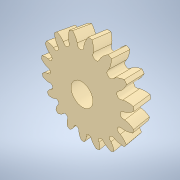
# Autodesk Inventor part: Промежуточная шестерня (малая)
Saved by Autodesk Inventor 2021.1 (Build 251245010, 245A)
## iProperties
Created: 2026-04-13
Part Number: Промежуточная шестерня (малая)
Material: Generic
Document SubType Name: Modeling
Designer: Андрей Тарасов
Density: 1 g/cm^3
Appearance: Default
Author: Андрей Тарасов
Autodesk Inventor part; units mm, degrees
ref_plane "YZ Plane" through (0, 0, 0) normal (1, 0, 0) x (0, 1, 0)
ref_plane "XZ Plane" through (0, 0, 0) normal (0, 1, 0) x (-1, 0, 0)
ref_plane "XY Plane" through (0, 0, 0) normal (0, 0, 1) x (1, 0, 0)
sketch "Sketch1" plane through (0, 0, 0) normal (0, 0, 1) x (1, 0, 0)
  spline S0 degree 3 poles (-2.4677, 16.4029) (-2.3891, 16.3117) (-2.2319, 16.1291) (-2.0115, 15.8426) (-1.8036, 15.5469) (-1.6113, 15.2408) (-1.4365, 14.9243) (-1.3084, 14.6515) (-1.219, 14.4277) (-1.1604, 14.2569) (-1.1092, 14.0833) (-1.0894, 13.9644) (-1.0796, 13.905) knots 0 0 0 0 0.036134 0.072267 0.1084 0.144533 0.180664 0.216793 0.23486 0.252926 0.270991 0.289046 0.289046 0.289046 0.289046
  spline S1 degree 3 poles (-1.0796, 13.905) (-1.0738, 13.8258) (-1.0651, 13.707) (-1.0412, 13.55) (-1.0167, 13.4334) (-0.9834, 13.319) (-0.9444, 13.2063) (-0.8925, 13.099) (-0.8339, 12.9952) (-0.7615, 12.9003) (-0.6769, 12.8161) (-0.5801, 12.7461) (-0.473, 12.6931) (-0.3574, 12.6608) (-0.1982, 12.6537) (0, 12.6626) (0.1982, 12.6537) (0.3574, 12.6608) (0.473, 12.6931) (0.5801, 12.7461) (0.6769, 12.8161) (0.7615, 12.9003) (0.8339, 12.9952) (0.8925, 13.099) (0.9444, 13.2063) (0.9834, 13.319) (1.0167, 13.4334) (1.0412, 13.55) (1.0651, 13.707) (1.0738, 13.8258) (1.0796, 13.905) knots 0 0 0 0 0.023807 0.035713 0.047621 0.059527 0.071434 0.083337 0.095237 0.107137 0.119035 0.130931 0.142823 0.154717 0.166615 0.19043 0.214245 0.226143 0.238037 0.249929 0.261825 0.273723 0.285623 0.297523 0.309426 0.321333 0.333239 0.345147 0.357054 0.38086 0.38086 0.38086 0.38086
  spline S2 degree 3 poles (1.0796, 13.905) (1.0894, 13.9644) (1.1092, 14.0833) (1.1604, 14.2569) (1.219, 14.4277) (1.3084, 14.6515) (1.4365, 14.9243) (1.6113, 15.2408) (1.8036, 15.5469) (2.0115, 15.8426) (2.2319, 16.1291) (2.3891, 16.3117) (2.4677, 16.4029) knots 0 0 0 0 0.018055 0.03612 0.054187 0.072254 0.108383 0.144514 0.180646 0.216779 0.252913 0.289046 0.289046 0.289046 0.289046
  circle A0 centre (0, 0) radius 12.659 construction
  circle A1 centre (0, 0) radius 13.946 construction
  circle A2 centre (0, 0) radius 14.841 construction
  circle A3 centre (0, 0) radius 16.5875
  spline S3 degree 3 poles (-6.0297, 12.5761) (-5.9957, 12.5043) (-5.9447, 12.3967) (-5.8658, 12.2589) (-5.8008, 12.159) (-5.7284, 12.0644) (-5.6513, 11.9734) (-5.5642, 11.8921) (-5.472, 11.8164) (-5.3702, 11.7541) (-5.2609, 11.7061) (-5.1453, 11.6758) (-5.0263, 11.6651) (-4.9069, 11.6767) (-4.7559, 11.7276) (-4.5743, 11.8075) (-4.3862, 11.8708) (-4.2403, 11.9349) (-4.1443, 12.0068) (-4.0635, 12.0949) (-3.9985, 12.1951) (-3.9501, 12.3043) (-3.9168, 12.4189) (-3.8996, 12.5369) (-3.89, 12.6557) (-3.8944, 12.7749) (-3.9046, 12.8935) (-3.9239, 13.0112) (-3.9584, 13.1662) (-3.9932, 13.2801) (-4.0164, 13.356) knots 0 0 0 0 0.023807 0.035713 0.047621 0.059527 0.071434 0.083337 0.095237 0.107137 0.119035 0.130931 0.142823 0.154717 0.166615 0.19043 0.214245 0.226143 0.238037 0.249929 0.261825 0.273723 0.285623 0.297523 0.309426 0.321333 0.333239 0.345147 0.357054 0.38086 0.38086 0.38086 0.38086
  spline S4 degree 3 poles (-4.0164, 13.356) (-4.0287, 13.415) (-4.0532, 13.533) (-4.0682, 13.7133) (-4.0752, 13.8938) (-4.0727, 14.1348) (-4.0517, 14.4354) (-4.0031, 14.7937) (-3.9343, 15.1486) (-3.8474, 15.4994) (-3.7453, 15.8462) (-3.6647, 16.0732) (-3.6243, 16.1867) knots 0 0 0 0 0.018055 0.03612 0.054187 0.072254 0.108383 0.144514 0.180646 0.216779 0.252913 0.289046 0.289046 0.289046 0.289046
  spline S5 degree 3 poles (-8.2265, 14.4038) (-8.1202, 14.3471) (-7.9077, 14.2337) (-7.5986, 14.0461) (-7.298, 13.8455) (-7.0081, 13.6295) (-6.7308, 13.3975) (-6.5128, 13.1895) (-6.3486, 13.0131) (-6.2322, 12.875) (-6.1218, 12.7316) (-6.0604, 12.6279) (-6.0297, 12.5761) knots 0 0 0 0 0.036134 0.072267 0.1084 0.144533 0.180664 0.216793 0.23486 0.252926 0.270991 0.289046 0.289046 0.289046 0.289046
  spline S6 degree 3 poles (-10.1655, 9.5486) (-10.1079, 9.494) (-10.0215, 9.4121) (-9.8981, 9.3121) (-9.8014, 9.2424) (-9.6997, 9.1804) (-9.595, 9.1233) (-9.4844, 9.079) (-9.3711, 9.0418) (-9.2536, 9.0204) (-9.1344, 9.0151) (-9.0156, 9.0287) (-8.9008, 9.0617) (-8.7936, 9.1156) (-8.6712, 9.2176) (-8.5307, 9.3578) (-8.3782, 9.4847) (-8.2654, 9.5972) (-8.2018, 9.699) (-8.1583, 9.8102) (-8.1339, 9.9272) (-8.1281, 10.0465) (-8.1385, 10.1654) (-8.1652, 10.2816) (-8.1991, 10.3959) (-8.2462, 10.5054) (-8.2986, 10.6124) (-8.3591, 10.7151) (-8.4473, 10.8472) (-8.5209, 10.9408) (-8.5699, 11.0032) knots 0 0 0 0 0.023807 0.035713 0.047621 0.059527 0.071434 0.083337 0.095237 0.107137 0.119035 0.130931 0.142823 0.154717 0.166615 0.19043 0.214245 0.226143 0.238037 0.249929 0.261825 0.273723 0.285623 0.297523 0.309426 0.321333 0.333239 0.345147 0.357054 0.38086 0.38086 0.38086 0.38086
  spline S7 degree 3 poles (-8.5699, 11.0032) (-8.6027, 11.0538) (-8.6682, 11.1549) (-8.7473, 11.3177) (-8.819, 11.4835) (-8.9037, 11.7091) (-8.9928, 11.997) (-9.0769, 12.3486) (-9.141, 12.7044) (-9.1866, 13.0629) (-9.2167, 13.4232) (-9.2235, 13.664) (-9.2269, 13.7844) knots 0 0 0 0 0.018055 0.03612 0.054187 0.072254 0.108383 0.144514 0.180646 0.216779 0.252913 0.289046 0.289046 0.289046 0.289046
  spline S8 degree 3 poles (-12.8743, 10.4594) (-12.7547, 10.4449) (-12.5155, 10.4159) (-12.1596, 10.3527) (-11.8067, 10.2742) (-11.4584, 10.1775) (-11.116, 10.0614) (-10.8376, 9.9461) (-10.6208, 9.841) (-10.4623, 9.7542) (-10.3076, 9.6604) (-10.2129, 9.5859) (-10.1655, 9.5486) knots 0 0 0 0 0.036134 0.072267 0.1084 0.144533 0.180664 0.216793 0.23486 0.252926 0.270991 0.289046 0.289046 0.289046 0.289046
  spline S9 degree 3 poles (-12.9285, 5.2316) (-12.855, 5.2015) (-12.7448, 5.1563) (-12.5936, 5.1077) (-12.4783, 5.0776) (-12.361, 5.0565) (-12.2428, 5.0411) (-12.1236, 5.0398) (-12.0046, 5.046) (-11.8873, 5.0685) (-11.7742, 5.1066) (-11.6684, 5.1622) (-11.5732, 5.2344) (-11.4928, 5.3234) (-11.4155, 5.4628) (-11.3351, 5.6442) (-11.2387, 5.8177) (-11.1741, 5.9633) (-11.1516, 6.0812) (-11.1513, 6.2007) (-11.1707, 6.3186) (-11.2085, 6.4318) (-11.2611, 6.539) (-11.3279, 6.6377) (-11.4009, 6.732) (-11.4844, 6.8171) (-11.5719, 6.8979) (-11.6654, 6.9718) (-11.7953, 7.0632) (-11.8977, 7.1239) (-11.9661, 7.1644) knots 0 0 0 0 0.023807 0.035713 0.047621 0.059527 0.071434 0.083337 0.095237 0.107137 0.119035 0.130931 0.142823 0.154717 0.166615 0.19043 0.214245 0.226143 0.238037 0.249929 0.261825 0.273723 0.285623 0.297523 0.309426 0.321333 0.333239 0.345147 0.357054 0.38086 0.38086 0.38086 0.38086
  spline S10 degree 3 poles (-11.9661, 7.1644) (-12.0148, 7.1997) (-12.1125, 7.2704) (-12.245, 7.3935) (-12.3718, 7.5222) (-12.5323, 7.702) (-12.7194, 7.9383) (-12.9247, 8.2358) (-13.113, 8.5444) (-13.2851, 8.8622) (-13.4433, 9.1873) (-13.5367, 9.4094) (-13.5833, 9.5204) knots 0 0 0 0 0.018055 0.03612 0.054187 0.072254 0.108383 0.144514 0.180646 0.216779 0.252913 0.289046 0.289046 0.289046 0.289046
  spline S11 degree 3 poles (-15.7833, 5.1024) (-15.6665, 5.1321) (-15.433, 5.1914) (-15.0783, 5.2611) (-14.7209, 5.3153) (-14.3612, 5.351) (-14, 5.3664) (-13.6987, 5.3595) (-13.4585, 5.3398) (-13.2794, 5.3161) (-13.1013, 5.2846) (-12.986, 5.2493) (-12.9285, 5.2316) knots 0 0 0 0 0.036134 0.072267 0.1084 0.144533 0.180664 0.216793 0.23486 0.252926 0.270991 0.289046 0.289046 0.289046 0.289046
  spline S12 degree 3 poles (-13.9453, 0.208) (-13.8659, 0.2065) (-13.7468, 0.2042) (-13.5883, 0.2134) (-13.4699, 0.2271) (-13.353, 0.2497) (-13.2371, 0.2781) (-13.1255, 0.3199) (-13.0167, 0.3687) (-12.9156, 0.4321) (-12.8238, 0.5085) (-12.7452, 0.5985) (-12.6826, 0.7002) (-12.6397, 0.8123) (-12.618, 0.9701) (-12.6086, 1.1684) (-12.5814, 1.3649) (-12.5738, 1.5241) (-12.5953, 1.6421) (-12.6382, 1.7536) (-12.6989, 1.8566) (-12.775, 1.9485) (-12.8628, 2.0294) (-12.9608, 2.0974) (-13.0629, 2.1589) (-13.1715, 2.2081) (-13.2823, 2.2519) (-13.3961, 2.287) (-13.5503, 2.3253) (-13.6678, 2.3449) (-13.7461, 2.3579) knots 0 0 0 0 0.023807 0.035713 0.047621 0.059527 0.071434 0.083337 0.095237 0.107137 0.119035 0.130931 0.142823 0.154717 0.166615 0.19043 0.214245 0.226143 0.238037 0.249929 0.261825 0.273723 0.285623 0.297523 0.309426 0.321333 0.333239 0.345147 0.357054 0.38086 0.38086 0.38086 0.38086
  spline S13 degree 3 poles (-13.7461, 2.3579) (-13.8043, 2.3733) (-13.9209, 2.4039) (-14.089, 2.4709) (-14.2537, 2.5451) (-14.4683, 2.6547) (-14.7281, 2.8074) (-15.0271, 3.0107) (-15.3141, 3.2304) (-15.5894, 3.4646) (-15.8544, 3.7106) (-16.0216, 3.884) (-16.1053, 3.9707) knots 0 0 0 0 0.018055 0.03612 0.054187 0.072254 0.108383 0.144514 0.180646 0.216779 0.252913 0.289046 0.289046 0.289046 0.289046
  spline S14 degree 3 poles (-16.5607, -0.9437) (-16.4625, -0.8739) (-16.2662, -0.7342) (-15.9606, -0.5411) (-15.647, -0.3614) (-15.3244, -0.1982) (-14.9932, -0.0534) (-14.7097, 0.049) (-14.4787, 0.1174) (-14.3031, 0.16) (-14.1256, 0.195) (-14.0054, 0.2037) (-13.9453, 0.208) knots 0 0 0 0 0.036134 0.072267 0.1084 0.144533 0.180664 0.216793 0.23486 0.252926 0.270991 0.289046 0.289046 0.289046 0.289046
  spline S15 degree 3 poles (-13.0788, -4.8436) (-13.0042, -4.8164) (-12.8923, -4.7755) (-12.7478, -4.7096) (-12.6423, -4.6541) (-12.5415, -4.5908) (-12.4437, -4.5225) (-12.3547, -4.4432) (-12.2709, -4.3584) (-12.1995, -4.2628) (-12.1416, -4.1584) (-12.1008, -4.046) (-12.0791, -3.9285) (-12.0796, -3.8086) (-12.1164, -3.6535) (-12.1792, -3.4653) (-12.2249, -3.2722) (-12.2753, -3.121) (-12.338, -3.0187) (-12.4182, -2.9302) (-12.5121, -2.8562) (-12.6163, -2.7979) (-12.7274, -2.7542) (-12.8432, -2.7262) (-12.9607, -2.7057) (-13.0797, -2.6991) (-13.1988, -2.6983) (-13.3177, -2.7066) (-13.4753, -2.7267) (-13.5919, -2.7508) (-13.6696, -2.7669) knots 0 0 0 0 0.023807 0.035713 0.047621 0.059527 0.071434 0.083337 0.095237 0.107137 0.119035 0.130931 0.142823 0.154717 0.166615 0.19043 0.214245 0.226143 0.238037 0.249929 0.261825 0.273723 0.285623 0.297523 0.309426 0.321333 0.333239 0.345147 0.357054 0.38086 0.38086 0.38086 0.38086
  spline S16 degree 3 poles (-13.6696, -2.7669) (-13.7295, -2.7737) (-13.8492, -2.7872) (-14.0302, -2.7855) (-14.2106, -2.7758) (-14.4503, -2.7511) (-14.7477, -2.7025) (-15.0999, -2.621) (-15.447, -2.5198) (-15.7883, -2.4009) (-16.1242, -2.2672) (-16.3428, -2.166) (-16.4521, -2.1153) knots 0 0 0 0 0.018055 0.03612 0.054187 0.072254 0.108383 0.144514 0.180646 0.216779 0.252913 0.289046 0.289046 0.289046 0.289046
  spline S17 degree 3 poles (-15.1014, -6.8624) (-15.0352, -6.7618) (-14.9026, -6.5606) (-14.6873, -6.2702) (-14.4598, -5.9894) (-14.218, -5.7206) (-13.9614, -5.4659) (-13.7341, -5.2681) (-13.5434, -5.1208) (-13.3951, -5.0176) (-13.2421, -4.9209) (-13.1332, -4.8694) (-13.0788, -4.8436) knots 0 0 0 0 0.036134 0.072267 0.1084 0.144533 0.180664 0.216793 0.23486 0.252926 0.270991 0.289046 0.289046 0.289046 0.289046
  spline S18 degree 3 poles (-10.4459, -9.2411) (-10.3862, -9.1888) (-10.2966, -9.1103) (-10.1857, -8.9966) (-10.1074, -8.9068) (-10.0362, -8.8113) (-9.9697, -8.7123) (-9.9154, -8.6062) (-9.8679, -8.4969) (-9.8358, -8.3819) (-9.8195, -8.2636) (-9.822, -8.1441) (-9.8443, -8.0267) (-9.8881, -7.915) (-9.9784, -7.7837) (-10.105, -7.6309) (-10.2173, -7.4673) (-10.3189, -7.3446) (-10.4144, -7.2719) (-10.5211, -7.2183) (-10.6354, -7.1832) (-10.7536, -7.1665) (-10.873, -7.1659) (-10.9911, -7.1817) (-11.108, -7.2049) (-11.2214, -7.2418) (-11.3328, -7.2841) (-11.4406, -7.3348) (-11.5803, -7.4104) (-11.6803, -7.475) (-11.747, -7.5181) knots 0 0 0 0 0.023807 0.035713 0.047621 0.059527 0.071434 0.083337 0.095237 0.107137 0.119035 0.130931 0.142823 0.154717 0.166615 0.19043 0.214245 0.226143 0.238037 0.249929 0.261825 0.273723 0.285623 0.297523 0.309426 0.321333 0.333239 0.345147 0.357054 0.38086 0.38086 0.38086 0.38086
  spline S19 degree 3 poles (-11.747, -7.5181) (-11.8004, -7.5461) (-11.9072, -7.6019) (-12.0765, -7.6657) (-12.2482, -7.7218) (-12.4807, -7.7854) (-12.7755, -7.8475) (-13.1334, -7.8988) (-13.4936, -7.9298) (-13.8548, -7.9421) (-14.2163, -7.9388) (-14.4567, -7.9234) (-14.577, -7.9157) knots 0 0 0 0 0.018055 0.03612 0.054187 0.072254 0.108383 0.144514 0.180646 0.216779 0.252913 0.289046 0.289046 0.289046 0.289046
  spline S20 degree 3 poles (-11.6027, -11.8543) (-11.5772, -11.7365) (-11.5263, -11.501) (-11.4305, -11.1525) (-11.3197, -10.8084) (-11.1914, -10.4705) (-11.0441, -10.1403) (-10.9036, -9.8737) (-10.7789, -9.6675) (-10.6779, -9.5177) (-10.5703, -9.3722) (-10.4873, -9.2848) (-10.4459, -9.2411) knots 0 0 0 0 0.036134 0.072267 0.1084 0.144533 0.180664 0.216793 0.23486 0.252926 0.270991 0.289046 0.289046 0.289046 0.289046
  spline S21 degree 3 poles (-6.4022, -12.3906) (-6.3654, -12.3202) (-6.3103, -12.2147) (-6.2479, -12.0686) (-6.2073, -11.9565) (-6.1755, -11.8418) (-6.1493, -11.7254) (-6.1369, -11.6069) (-6.1321, -11.4878) (-6.1437, -11.3689) (-6.1712, -11.2528) (-6.2168, -11.1423) (-6.28, -11.0409) (-6.3611, -10.9526) (-6.4928, -10.8627) (-6.666, -10.7659) (-6.8298, -10.654) (-6.9689, -10.5762) (-7.0842, -10.5429) (-7.2031, -10.5316) (-7.3223, -10.5401) (-7.4386, -10.5672) (-7.5501, -10.6098) (-7.6546, -10.6672) (-7.7552, -10.7311) (-7.8477, -10.8064) (-7.9362, -10.8861) (-8.0184, -10.9723) (-8.1214, -11.0933) (-8.1913, -11.1897) (-8.2379, -11.254) knots 0 0 0 0 0.023807 0.035713 0.047621 0.059527 0.071434 0.083337 0.095237 0.107137 0.119035 0.130931 0.142823 0.154717 0.166615 0.19043 0.214245 0.226143 0.238037 0.249929 0.261825 0.273723 0.285623 0.297523 0.309426 0.321333 0.333239 0.345147 0.357054 0.38086 0.38086 0.38086 0.38086
  spline S22 degree 3 poles (-8.2379, -11.254) (-8.2776, -11.2993) (-8.357, -11.39) (-8.4918, -11.5106) (-8.6317, -11.625) (-8.8255, -11.7682) (-9.078, -11.9326) (-9.3932, -12.1097) (-9.7178, -12.2687) (-10.0502, -12.4107) (-10.3885, -12.5383) (-10.6183, -12.6107) (-10.7331, -12.647) knots 0 0 0 0 0.018055 0.03612 0.054187 0.072254 0.108383 0.144514 0.180646 0.216779 0.252913 0.289046 0.289046 0.289046 0.289046
  spline S23 degree 3 poles (-6.5369, -15.2451) (-6.5557, -15.1262) (-6.5933, -14.8882) (-6.6299, -14.5285) (-6.6509, -14.1677) (-6.6533, -13.8062) (-6.6353, -13.4451) (-6.6006, -13.1458) (-6.5588, -12.9084) (-6.5187, -12.7323) (-6.4709, -12.5578) (-6.4251, -12.4463) (-6.4022, -12.3906) knots 0 0 0 0 0.036134 0.072267 0.1084 0.144533 0.180664 0.216793 0.23486 0.252926 0.270991 0.289046 0.289046 0.289046 0.289046
  spline S24 degree 3 poles (-1.4939, -13.8666) (-1.485, -13.7877) (-1.4717, -13.6694) (-1.4663, -13.5106) (-1.469, -13.3915) (-1.4807, -13.2729) (-1.4983, -13.155) (-1.5296, -13.04) (-1.5681, -12.9272) (-1.6219, -12.8206) (-1.6895, -12.7222) (-1.7719, -12.6356) (-1.8675, -12.5639) (-1.9751, -12.5109) (-2.1302, -12.4747) (-2.3267, -12.447) (-2.52, -12.4018) (-2.6777, -12.3795) (-2.7973, -12.3901) (-2.9123, -12.4225) (-3.0203, -12.4735) (-3.1189, -12.5408) (-3.2076, -12.6207) (-3.2843, -12.712) (-3.355, -12.8079) (-3.414, -12.9116) (-3.4678, -13.0178) (-3.5133, -13.128) (-3.5656, -13.2779) (-3.596, -13.3931) (-3.6162, -13.4699) knots 0 0 0 0 0.023807 0.035713 0.047621 0.059527 0.071434 0.083337 0.095237 0.107137 0.119035 0.130931 0.142823 0.154717 0.166615 0.19043 0.214245 0.226143 0.238037 0.249929 0.261825 0.273723 0.285623 0.297523 0.309426 0.321333 0.333239 0.345147 0.357054 0.38086 0.38086 0.38086 0.38086
  spline S25 degree 3 poles (-3.6162, -13.4699) (-3.6368, -13.5265) (-3.6781, -13.6397) (-3.7603, -13.8009) (-3.8494, -13.9581) (-3.9784, -14.1616) (-4.1544, -14.4062) (-4.3843, -14.6852) (-4.6296, -14.9507) (-4.8883, -15.2032) (-5.1576, -15.4444) (-5.3457, -15.5949) (-5.4397, -15.6702) knots 0 0 0 0 0.018055 0.03612 0.054187 0.072254 0.108383 0.144514 0.180646 0.216779 0.252913 0.289046 0.289046 0.289046 0.289046
  spline S26 degree 3 poles (-0.5883, -16.5771) (-0.6488, -16.4729) (-0.7698, -16.2646) (-0.9339, -15.9424) (-1.0838, -15.6136) (-1.2166, -15.2773) (-1.3303, -14.9341) (-1.406, -14.6425) (-1.4528, -14.4061) (-1.4791, -14.2273) (-1.4975, -14.0473) (-1.4951, -13.9268) (-1.4939, -13.8666) knots 0 0 0 0 0.036134 0.072267 0.1084 0.144533 0.180664 0.216793 0.23486 0.252926 0.270991 0.289046 0.289046 0.289046 0.289046
  spline S27 degree 3 poles (3.6162, -13.4699) (3.596, -13.3931) (3.5656, -13.2779) (3.5133, -13.128) (3.4678, -13.0178) (3.414, -12.9116) (3.355, -12.8079) (3.2843, -12.712) (3.2076, -12.6207) (3.1189, -12.5408) (3.0203, -12.4735) (2.9123, -12.4225) (2.7973, -12.3901) (2.6777, -12.3795) (2.52, -12.4018) (2.3267, -12.447) (2.1302, -12.4747) (1.9751, -12.5109) (1.8675, -12.5639) (1.7719, -12.6356) (1.6895, -12.7222) (1.6219, -12.8206) (1.5681, -12.9272) (1.5296, -13.04) (1.4983, -13.155) (1.4807, -13.2729) (1.469, -13.3915) (1.4663, -13.5106) (1.4717, -13.6694) (1.485, -13.7877) (1.4939, -13.8666) knots 0 0 0 0 0.023807 0.035713 0.047621 0.059527 0.071434 0.083337 0.095237 0.107137 0.119035 0.130931 0.142823 0.154717 0.166615 0.19043 0.214245 0.226143 0.238037 0.249929 0.261825 0.273723 0.285623 0.297523 0.309426 0.321333 0.333239 0.345147 0.357054 0.38086 0.38086 0.38086 0.38086
  spline S28 degree 3 poles (1.4939, -13.8666) (1.4951, -13.9268) (1.4975, -14.0473) (1.4791, -14.2273) (1.4528, -14.4061) (1.406, -14.6425) (1.3303, -14.9341) (1.2166, -15.2773) (1.0838, -15.6136) (0.9339, -15.9424) (0.7698, -16.2646) (0.6488, -16.4729) (0.5883, -16.5771) knots 0 0 0 0 0.018055 0.03612 0.054187 0.072254 0.108383 0.144514 0.180646 0.216779 0.252913 0.289046 0.289046 0.289046 0.289046
  spline S29 degree 3 poles (5.4397, -15.6702) (5.3457, -15.5949) (5.1576, -15.4444) (4.8883, -15.2032) (4.6296, -14.9507) (4.3843, -14.6852) (4.1544, -14.4062) (3.9784, -14.1616) (3.8494, -13.9581) (3.7603, -13.8009) (3.6781, -13.6397) (3.6368, -13.5265) (3.6162, -13.4699) knots 0 0 0 0 0.036134 0.072267 0.1084 0.144533 0.180664 0.216793 0.23486 0.252926 0.270991 0.289046 0.289046 0.289046 0.289046
  spline S30 degree 3 poles (8.2379, -11.254) (8.1913, -11.1897) (8.1214, -11.0933) (8.0184, -10.9723) (7.9362, -10.8861) (7.8477, -10.8064) (7.7552, -10.7311) (7.6546, -10.6672) (7.5501, -10.6098) (7.4386, -10.5672) (7.3223, -10.5401) (7.2031, -10.5316) (7.0842, -10.5429) (6.9689, -10.5762) (6.8298, -10.654) (6.666, -10.7659) (6.4928, -10.8627) (6.3611, -10.9526) (6.28, -11.0409) (6.2168, -11.1423) (6.1712, -11.2528) (6.1437, -11.3689) (6.1321, -11.4878) (6.1369, -11.6069) (6.1493, -11.7254) (6.1755, -11.8418) (6.2073, -11.9565) (6.2479, -12.0686) (6.3103, -12.2147) (6.3654, -12.3202) (6.4022, -12.3906) knots 0 0 0 0 0.023807 0.035713 0.047621 0.059527 0.071434 0.083337 0.095237 0.107137 0.119035 0.130931 0.142823 0.154717 0.166615 0.19043 0.214245 0.226143 0.238037 0.249929 0.261825 0.273723 0.285623 0.297523 0.309426 0.321333 0.333239 0.345147 0.357054 0.38086 0.38086 0.38086 0.38086
  spline S31 degree 3 poles (6.4022, -12.3906) (6.4251, -12.4463) (6.4709, -12.5578) (6.5187, -12.7323) (6.5588, -12.9084) (6.6006, -13.1458) (6.6353, -13.4451) (6.6533, -13.8062) (6.6509, -14.1677) (6.6299, -14.5285) (6.5933, -14.8882) (6.5557, -15.1262) (6.5369, -15.2451) knots 0 0 0 0 0.018055 0.03612 0.054187 0.072254 0.108383 0.144514 0.180646 0.216779 0.252913 0.289046 0.289046 0.289046 0.289046
  spline S32 degree 3 poles (10.7331, -12.647) (10.6183, -12.6107) (10.3885, -12.5383) (10.0502, -12.4107) (9.7178, -12.2687) (9.3932, -12.1097) (9.078, -11.9326) (8.8255, -11.7682) (8.6317, -11.625) (8.4918, -11.5106) (8.357, -11.39) (8.2776, -11.2993) (8.2379, -11.254) knots 0 0 0 0 0.036134 0.072267 0.1084 0.144533 0.180664 0.216793 0.23486 0.252926 0.270991 0.289046 0.289046 0.289046 0.289046
  spline S33 degree 3 poles (11.747, -7.5181) (11.6803, -7.475) (11.5803, -7.4104) (11.4406, -7.3348) (11.3328, -7.2841) (11.2214, -7.2418) (11.108, -7.2049) (10.9911, -7.1817) (10.873, -7.1659) (10.7536, -7.1665) (10.6354, -7.1832) (10.5211, -7.2183) (10.4144, -7.2719) (10.3189, -7.3446) (10.2173, -7.4673) (10.105, -7.6309) (9.9784, -7.7837) (9.8881, -7.915) (9.8443, -8.0267) (9.822, -8.1441) (9.8195, -8.2636) (9.8358, -8.3819) (9.8679, -8.4969) (9.9154, -8.6062) (9.9697, -8.7123) (10.0362, -8.8113) (10.1074, -8.9068) (10.1857, -8.9966) (10.2966, -9.1103) (10.3862, -9.1888) (10.4459, -9.2411) knots 0 0 0 0 0.023807 0.035713 0.047621 0.059527 0.071434 0.083337 0.095237 0.107137 0.119035 0.130931 0.142823 0.154717 0.166615 0.19043 0.214245 0.226143 0.238037 0.249929 0.261825 0.273723 0.285623 0.297523 0.309426 0.321333 0.333239 0.345147 0.357054 0.38086 0.38086 0.38086 0.38086
  spline S34 degree 3 poles (10.4459, -9.2411) (10.4873, -9.2848) (10.5703, -9.3722) (10.6779, -9.5177) (10.7789, -9.6675) (10.9036, -9.8737) (11.0441, -10.1403) (11.1914, -10.4705) (11.3197, -10.8084) (11.4305, -11.1525) (11.5263, -11.501) (11.5772, -11.7365) (11.6027, -11.8543) knots 0 0 0 0 0.018055 0.03612 0.054187 0.072254 0.108383 0.144514 0.180646 0.216779 0.252913 0.289046 0.289046 0.289046 0.289046
  spline S35 degree 3 poles (14.577, -7.9157) (14.4567, -7.9234) (14.2163, -7.9388) (13.8548, -7.9421) (13.4936, -7.9298) (13.1334, -7.8988) (12.7755, -7.8475) (12.4807, -7.7854) (12.2482, -7.7218) (12.0765, -7.6657) (11.9072, -7.6019) (11.8004, -7.5461) (11.747, -7.5181) knots 0 0 0 0 0.036134 0.072267 0.1084 0.144533 0.180664 0.216793 0.23486 0.252926 0.270991 0.289046 0.289046 0.289046 0.289046
  spline S36 degree 3 poles (13.6696, -2.7669) (13.5919, -2.7508) (13.4753, -2.7267) (13.3177, -2.7066) (13.1988, -2.6983) (13.0797, -2.6991) (12.9607, -2.7057) (12.8432, -2.7262) (12.7274, -2.7542) (12.6163, -2.7979) (12.5121, -2.8562) (12.4182, -2.9302) (12.338, -3.0187) (12.2753, -3.121) (12.2249, -3.2722) (12.1792, -3.4653) (12.1164, -3.6535) (12.0796, -3.8086) (12.0791, -3.9285) (12.1008, -4.046) (12.1416, -4.1584) (12.1995, -4.2628) (12.2709, -4.3584) (12.3547, -4.4432) (12.4437, -4.5225) (12.5415, -4.5908) (12.6423, -4.6541) (12.7478, -4.7096) (12.8923, -4.7755) (13.0042, -4.8164) (13.0788, -4.8436) knots 0 0 0 0 0.023807 0.035713 0.047621 0.059527 0.071434 0.083337 0.095237 0.107137 0.119035 0.130931 0.142823 0.154717 0.166615 0.19043 0.214245 0.226143 0.238037 0.249929 0.261825 0.273723 0.285623 0.297523 0.309426 0.321333 0.333239 0.345147 0.357054 0.38086 0.38086 0.38086 0.38086
  spline S37 degree 3 poles (13.0788, -4.8436) (13.1332, -4.8694) (13.2421, -4.9209) (13.3951, -5.0176) (13.5434, -5.1208) (13.7341, -5.2681) (13.9614, -5.4659) (14.218, -5.7206) (14.4598, -5.9894) (14.6873, -6.2702) (14.9026, -6.5606) (15.0352, -6.7618) (15.1014, -6.8624) knots 0 0 0 0 0.018055 0.03612 0.054187 0.072254 0.108383 0.144514 0.180646 0.216779 0.252913 0.289046 0.289046 0.289046 0.289046
  spline S38 degree 3 poles (16.4521, -2.1153) (16.3428, -2.166) (16.1242, -2.2672) (15.7883, -2.4009) (15.447, -2.5198) (15.0999, -2.621) (14.7477, -2.7025) (14.4503, -2.7511) (14.2106, -2.7758) (14.0302, -2.7855) (13.8492, -2.7872) (13.7295, -2.7737) (13.6696, -2.7669) knots 0 0 0 0 0.036134 0.072267 0.1084 0.144533 0.180664 0.216793 0.23486 0.252926 0.270991 0.289046 0.289046 0.289046 0.289046
  spline S39 degree 3 poles (13.7461, 2.3579) (13.6678, 2.3449) (13.5503, 2.3253) (13.3961, 2.287) (13.2823, 2.2519) (13.1715, 2.2081) (13.0629, 2.1589) (12.9608, 2.0974) (12.8628, 2.0294) (12.775, 1.9485) (12.6989, 1.8566) (12.6382, 1.7536) (12.5953, 1.6421) (12.5738, 1.5241) (12.5814, 1.3649) (12.6086, 1.1684) (12.618, 0.9701) (12.6397, 0.8123) (12.6826, 0.7002) (12.7452, 0.5985) (12.8238, 0.5085) (12.9156, 0.4321) (13.0167, 0.3687) (13.1255, 0.3199) (13.2371, 0.2781) (13.353, 0.2497) (13.4699, 0.2271) (13.5883, 0.2134) (13.7468, 0.2042) (13.8659, 0.2065) (13.9453, 0.208) knots 0 0 0 0 0.023807 0.035713 0.047621 0.059527 0.071434 0.083337 0.095237 0.107137 0.119035 0.130931 0.142823 0.154717 0.166615 0.19043 0.214245 0.226143 0.238037 0.249929 0.261825 0.273723 0.285623 0.297523 0.309426 0.321333 0.333239 0.345147 0.357054 0.38086 0.38086 0.38086 0.38086
  spline S40 degree 3 poles (13.9453, 0.208) (14.0054, 0.2037) (14.1256, 0.195) (14.3031, 0.16) (14.4787, 0.1174) (14.7097, 0.049) (14.9932, -0.0534) (15.3244, -0.1982) (15.647, -0.3614) (15.9606, -0.5411) (16.2662, -0.7342) (16.4625, -0.8739) (16.5607, -0.9437) knots 0 0 0 0 0.018055 0.03612 0.054187 0.072254 0.108383 0.144514 0.180646 0.216779 0.252913 0.289046 0.289046 0.289046 0.289046
  spline S41 degree 3 poles (16.1053, 3.9707) (16.0216, 3.884) (15.8544, 3.7106) (15.5894, 3.4646) (15.3141, 3.2304) (15.0271, 3.0107) (14.7281, 2.8074) (14.4683, 2.6547) (14.2537, 2.5451) (14.089, 2.4709) (13.9209, 2.4039) (13.8043, 2.3733) (13.7461, 2.3579) knots 0 0 0 0 0.036134 0.072267 0.1084 0.144533 0.180664 0.216793 0.23486 0.252926 0.270991 0.289046 0.289046 0.289046 0.289046
  spline S42 degree 3 poles (11.9661, 7.1644) (11.8977, 7.1239) (11.7953, 7.0632) (11.6654, 6.9718) (11.5719, 6.8979) (11.4844, 6.8171) (11.4009, 6.732) (11.3279, 6.6377) (11.2611, 6.539) (11.2085, 6.4318) (11.1707, 6.3186) (11.1513, 6.2007) (11.1516, 6.0812) (11.1741, 5.9633) (11.2387, 5.8177) (11.3351, 5.6442) (11.4155, 5.4628) (11.4928, 5.3234) (11.5732, 5.2344) (11.6684, 5.1622) (11.7742, 5.1066) (11.8873, 5.0685) (12.0046, 5.046) (12.1236, 5.0398) (12.2428, 5.0411) (12.361, 5.0565) (12.4783, 5.0776) (12.5936, 5.1077) (12.7448, 5.1563) (12.855, 5.2015) (12.9285, 5.2316) knots 0 0 0 0 0.023807 0.035713 0.047621 0.059527 0.071434 0.083337 0.095237 0.107137 0.119035 0.130931 0.142823 0.154717 0.166615 0.19043 0.214245 0.226143 0.238037 0.249929 0.261825 0.273723 0.285623 0.297523 0.309426 0.321333 0.333239 0.345147 0.357054 0.38086 0.38086 0.38086 0.38086
  spline S43 degree 3 poles (12.9285, 5.2316) (12.986, 5.2493) (13.1013, 5.2846) (13.2794, 5.3161) (13.4585, 5.3398) (13.6987, 5.3595) (14, 5.3664) (14.3612, 5.351) (14.7209, 5.3153) (15.0783, 5.2611) (15.433, 5.1914) (15.6665, 5.1321) (15.7833, 5.1024) knots 0 0 0 0 0.018055 0.03612 0.054187 0.072254 0.108383 0.144514 0.180646 0.216779 0.252913 0.289046 0.289046 0.289046 0.289046
  spline S44 degree 3 poles (13.5833, 9.5204) (13.5367, 9.4094) (13.4433, 9.1873) (13.2851, 8.8622) (13.113, 8.5444) (12.9247, 8.2358) (12.7194, 7.9383) (12.5323, 7.702) (12.3718, 7.5222) (12.245, 7.3935) (12.1125, 7.2704) (12.0148, 7.1997) (11.9661, 7.1644) knots 0 0 0 0 0.036134 0.072267 0.1084 0.144533 0.180664 0.216793 0.23486 0.252926 0.270991 0.289046 0.289046 0.289046 0.289046
  spline S45 degree 3 poles (8.5699, 11.0032) (8.5209, 10.9408) (8.4473, 10.8472) (8.3591, 10.7151) (8.2986, 10.6124) (8.2462, 10.5054) (8.1991, 10.3959) (8.1652, 10.2816) (8.1385, 10.1654) (8.1281, 10.0465) (8.1339, 9.9272) (8.1583, 9.8102) (8.2018, 9.699) (8.2654, 9.5972) (8.3782, 9.4847) (8.5307, 9.3578) (8.6712, 9.2176) (8.7936, 9.1156) (8.9008, 9.0617) (9.0156, 9.0287) (9.1344, 9.0151) (9.2536, 9.0204) (9.3711, 9.0418) (9.4844, 9.079) (9.595, 9.1233) (9.6997, 9.1804) (9.8014, 9.2424) (9.8981, 9.3121) (10.0215, 9.4121) (10.1079, 9.494) (10.1655, 9.5486) knots 0 0 0 0 0.023807 0.035713 0.047621 0.059527 0.071434 0.083337 0.095237 0.107137 0.119035 0.130931 0.142823 0.154717 0.166615 0.19043 0.214245 0.226143 0.238037 0.249929 0.261825 0.273723 0.285623 0.297523 0.309426 0.321333 0.333239 0.345147 0.357054 0.38086 0.38086 0.38086 0.38086
  spline S46 degree 3 poles (10.1655, 9.5486) (10.2129, 9.5859) (10.3076, 9.6604) (10.4623, 9.7542) (10.6208, 9.841) (10.8376, 9.9461) (11.116, 10.0614) (11.4584, 10.1775) (11.8067, 10.2742) (12.1596, 10.3527) (12.5155, 10.4159) (12.7547, 10.4449) (12.8743, 10.4594) knots 0 0 0 0 0.018055 0.03612 0.054187 0.072254 0.108383 0.144514 0.180646 0.216779 0.252913 0.289046 0.289046 0.289046 0.289046
  spline S47 degree 3 poles (9.2269, 13.7844) (9.2235, 13.664) (9.2167, 13.4232) (9.1866, 13.0629) (9.141, 12.7044) (9.0769, 12.3486) (8.9928, 11.997) (8.9037, 11.7091) (8.819, 11.4835) (8.7473, 11.3177) (8.6682, 11.1549) (8.6027, 11.0538) (8.5699, 11.0032) knots 0 0 0 0 0.036134 0.072267 0.1084 0.144533 0.180664 0.216793 0.23486 0.252926 0.270991 0.289046 0.289046 0.289046 0.289046
  spline S48 degree 3 poles (4.0164, 13.356) (3.9932, 13.2801) (3.9584, 13.1662) (3.9239, 13.0112) (3.9046, 12.8935) (3.8944, 12.7749) (3.89, 12.6557) (3.8996, 12.5369) (3.9168, 12.4189) (3.9501, 12.3043) (3.9985, 12.1951) (4.0635, 12.0949) (4.1443, 12.0068) (4.2403, 11.9349) (4.3862, 11.8708) (4.5743, 11.8075) (4.7559, 11.7276) (4.9069, 11.6767) (5.0263, 11.6651) (5.1453, 11.6758) (5.2609, 11.7061) (5.3702, 11.7541) (5.472, 11.8164) (5.5642, 11.8921) (5.6513, 11.9734) (5.7284, 12.0644) (5.8008, 12.159) (5.8658, 12.2589) (5.9447, 12.3967) (5.9957, 12.5043) (6.0297, 12.5761) knots 0 0 0 0 0.023807 0.035713 0.047621 0.059527 0.071434 0.083337 0.095237 0.107137 0.119035 0.130931 0.142823 0.154717 0.166615 0.19043 0.214245 0.226143 0.238037 0.249929 0.261825 0.273723 0.285623 0.297523 0.309426 0.321333 0.333239 0.345147 0.357054 0.38086 0.38086 0.38086 0.38086
  spline S49 degree 3 poles (6.0297, 12.5761) (6.0604, 12.6279) (6.1218, 12.7316) (6.2322, 12.875) (6.3486, 13.0131) (6.5128, 13.1895) (6.7308, 13.3975) (7.0081, 13.6295) (7.298, 13.8455) (7.5986, 14.0461) (7.9077, 14.2337) (8.1202, 14.3471) (8.2265, 14.4038) knots 0 0 0 0 0.018055 0.03612 0.054187 0.072254 0.108383 0.144514 0.180646 0.216779 0.252913 0.289046 0.289046 0.289046 0.289046
  spline S50 degree 3 poles (3.6243, 16.1867) (3.6647, 16.0732) (3.7453, 15.8462) (3.8474, 15.4994) (3.9343, 15.1486) (4.0031, 14.7937) (4.0517, 14.4354) (4.0727, 14.1348) (4.0752, 13.8938) (4.0682, 13.7133) (4.0532, 13.533) (4.0287, 13.415) (4.0164, 13.356) knots 0 0 0 0 0.036134 0.072267 0.1084 0.144533 0.180664 0.216793 0.23486 0.252926 0.270991 0.289046 0.289046 0.289046 0.289046
  circle A4 centre (0, 0) radius 4
  point P0 (-2.2345, 16.127)
  point P1 (-2.0136, 15.841)
  point P2 (-1.8062, 15.5451)
  point P3 (-1.6142, 15.239)
  point P4 (-1.44, 14.9225)
  point P5 (-1.2872, 14.5951)
  point P6 (-1.2204, 14.4272)
  point P7 (-1.1616, 14.2564)
  point P8 (-1.1128, 14.0825)
  point P9 (-1.0581, 13.6679)
  point P10 (-1.0401, 13.5502)
  point P11 (-1.0153, 13.4338)
  point P12 (-0.9824, 13.3193)
  point P13 (-0.9423, 13.2072)
  point P14 (-0.8914, 13.0996)
  point P15 (-0.8316, 12.9967)
  point P16 (-0.7595, 12.9021)
  point P17 (-0.6749, 12.8184)
  point P18 (-0.5783, 12.7489)
  point P19 (-0.4716, 12.6966)
  point P20 (-0.3568, 12.6653)
  point P21 (-0.2381, 12.6566)
  point P22 (0, 12.659)
  point P23 (0.2381, 12.6566)
  point P24 (0.3568, 12.6653)
  point P25 (0.4716, 12.6966)
  point P26 (0.5783, 12.7489)
  point P27 (0.6749, 12.8184)
  point P28 (0.7595, 12.9021)
  point P29 (0.8316, 12.9967)
  point P30 (0.8914, 13.0996)
  point P31 (0.9423, 13.2072)
  point P32 (0.9824, 13.3193)
  point P33 (1.0153, 13.4338)
  point P34 (1.0401, 13.5502)
  point P35 (1.0581, 13.6679)
  point P36 (1.1128, 14.0825)
  point P37 (1.1616, 14.2564)
  point P38 (1.2204, 14.4272)
  point P39 (1.2872, 14.5951)
  point P40 (1.44, 14.9225)
  point P41 (1.6142, 15.239)
  point P42 (1.8062, 15.5451)
  point P43 (2.0136, 15.841)
  point P44 (2.2345, 16.127)
  point P45 (-4.7942, 11.7159)
  point P46 (-4.573, 11.8042)
  point P47 (-4.2425, 11.9389)
  point P48 (-4.9079, 11.6811)
  point P49 (-4.1468, 12.0095)
  point P50 (-5.1447, 11.6791)
  point P51 (-4.0662, 12.0969)
  point P52 (-5.2598, 11.709)
  point P53 (-4.0013, 12.1966)
  point P54 (-5.3689, 11.7565)
  point P55 (-3.9526, 12.3052)
  point P56 (-5.4704, 11.8187)
  point P57 (-3.9195, 12.4195)
  point P58 (-3.9009, 12.537)
  point P59 (-5.5633, 11.893)
  point P60 (-5.6496, 11.975)
  point P61 (-3.8924, 12.6558)
  point P62 (-5.7276, 12.065)
  point P63 (-3.8954, 12.7748)
  point P64 (-5.7995, 12.1599)
  point P65 (-5.8648, 12.2595)
  point P66 (-5.9241, 12.3627)
  point P67 (-5.0262, 11.6688)
  point P68 (-4.35, 11.888)
  point P69 (-3.9061, 12.8934)
  point P70 (-3.925, 13.0109)
  point P71 (-3.9508, 13.1272)
  point P72 (-4.0496, 13.5335)
  point P73 (-4.0668, 13.7133)
  point P74 (-4.0737, 13.8939)
  point P75 (-4.0721, 14.0745)
  point P76 (-4.0478, 14.435)
  point P77 (-3.9998, 14.7931)
  point P78 (-3.9313, 15.1479)
  point P79 (-3.8449, 15.4987)
  point P80 (-3.7422, 15.8451)
  point P81 (-7.9093, 14.2308)
  point P82 (-7.6, 14.0439)
  point P83 (-7.2998, 13.8429)
  point P84 (-7.0102, 13.6268)
  point P85 (-6.7334, 13.3946)
  point P86 (-6.4726, 13.1446)
  point P87 (-6.3497, 13.0121)
  point P88 (-6.2332, 12.8741)
  point P89 (-6.1248, 12.7295)
  point P90 (-8.7027, 9.1929)
  point P91 (-8.5283, 9.3551)
  point P92 (-8.2689, 9.6001)
  point P93 (-8.7962, 9.1194)
  point P94 (-8.2051, 9.7006)
  point P95 (-9.0163, 9.0319)
  point P96 (-8.1615, 9.8112)
  point P97 (-9.1345, 9.0183)
  point P98 (-8.137, 9.9276)
  point P99 (-9.2533, 9.0231)
  point P100 (-8.1308, 10.0464)
  point P101 (-9.3704, 9.0444)
  point P102 (-8.1412, 10.165)
  point P103 (-8.1664, 10.2813)
  point P104 (-9.4839, 9.0802)
  point P105 (-9.594, 9.1254)
  point P106 (-8.2013, 10.3951)
  point P107 (-9.6992, 9.1812)
  point P108 (-8.2471, 10.505)
  point P109 (-9.8005, 9.2437)
  point P110 (-9.8974, 9.313)
  point P111 (-9.99, 9.3879)
  point P112 (-8.9021, 9.0652)
  point P113 (-8.3507, 9.5138)
  point P114 (-8.3, 10.6116)
  point P115 (-8.36, 10.7145)
  point P116 (-8.4261, 10.8136)
  point P117 (-8.665, 11.1567)
  point P118 (-8.746, 11.3182)
  point P119 (-8.8176, 11.484)
  point P120 (-8.8814, 11.6531)
  point P121 (-8.989, 11.998)
  point P122 (-9.0735, 12.3493)
  point P123 (-9.1379, 12.7048)
  point P124 (-9.184, 13.0632)
  point P125 (-9.2134, 13.4233)
  point P126 (-12.516, 10.4126)
  point P127 (-12.1601, 10.3501)
  point P128 (-11.8075, 10.2712)
  point P129 (-11.4594, 10.1743)
  point P130 (-11.1174, 10.0577)
  point P131 (-10.7839, 9.9188)
  point P132 (-10.6215, 9.8396)
  point P133 (-10.4629, 9.753)
  point P134 (-10.3097, 9.6574)
  point P135 (-11.4359, 5.4284)
  point P136 (-11.3319, 5.6426)
  point P137 (-11.1785, 5.9648)
  point P138 (-11.4965, 5.326)
  point P139 (-11.1553, 6.0815)
  point P140 (-11.6701, 5.165)
  point P141 (-11.1546, 6.2004)
  point P142 (-11.7754, 5.1096)
  point P143 (-11.1738, 6.3178)
  point P144 (-11.888, 5.0711)
  point P145 (-11.211, 6.4308)
  point P146 (-12.0049, 5.0487)
  point P147 (-11.2635, 6.5376)
  point P148 (-11.3289, 6.637)
  point P149 (-12.1236, 5.041)
  point P150 (-12.2426, 5.0435)
  point P151 (-11.4026, 6.7305)
  point P152 (-12.3609, 5.0575)
  point P153 (-11.485, 6.8164)
  point P154 (-12.4779, 5.0791)
  point P155 (-12.5933, 5.1088)
  point P156 (-12.7067, 5.1451)
  point P157 (-11.5757, 5.2372)
  point P158 (-11.2236, 5.8547)
  point P159 (-11.5729, 6.8968)
  point P160 (-11.666, 6.9709)
  point P161 (-11.7634, 7.0395)
  point P162 (-12.1101, 7.2732)
  point P163 (-12.244, 7.3945)
  point P164 (-12.3707, 7.5233)
  point P165 (-12.4913, 7.6578)
  point P166 (-12.7162, 7.9406)
  point P167 (-12.9219, 8.2376)
  point P168 (-13.1103, 8.5459)
  point P169 (-13.2828, 8.8634)
  point P170 (-13.4403, 9.1886)
  point P171 (-15.4323, 5.1882)
  point P172 (-15.0778, 5.2585)
  point P173 (-14.7205, 5.3122)
  point P174 (-14.3609, 5.3476)
  point P175 (-13.9999, 5.3624)
  point P176 (-13.6388, 5.3534)
  point P177 (-13.4587, 5.3383)
  point P178 (-13.2796, 5.3148)
  point P179 (-13.1021, 5.281)
  point P180 (-12.6246, 0.9307)
  point P181 (-12.605, 1.168)
  point P182 (-12.5783, 1.5239)
  point P183 (-12.6442, 0.8133)
  point P184 (-12.5989, 1.641)
  point P185 (-12.7479, 0.6004)
  point P186 (-12.6412, 1.7522)
  point P187 (-12.826, 0.5107)
  point P188 (-12.7015, 1.8547)
  point P189 (-12.9171, 0.4342)
  point P190 (-12.777, 1.9467)
  point P191 (-13.018, 0.3711)
  point P192 (-12.8645, 2.0273)
  point P193 (-12.9615, 2.0963)
  point P194 (-13.126, 0.3211)
  point P195 (-13.2378, 0.2804)
  point P196 (-13.0639, 2.1569)
  point P197 (-13.3531, 0.2507)
  point P198 (-13.1718, 2.2072)
  point P199 (-13.4701, 0.2286)
  dimension "d4" = 360
  dimension "d6" = 8
  constraints: 4 centre point, 1 coincident, 1809 other
  measures "d6" diameter of A4
extrude "Выдавливание1" add sketch "Sketch1" against normal blind 6 contours S0 S1 S2 A3 S50 S48 S49 S47 S45 S46 S44 S42 S43 S41 S39 S40 S38 S36 S37 S35 S33 S34 S32 S30 S31 S29 S27 S28 S26 S24 S25 S23 S21 S22 S20 S18 S19 S17 S15 S16 S14 S12 S13 S11 S9 S10 S8 S6 S7 S5 S3 S4
equation "\"d0\" = Ширина_грани"
equation "\"Модуль\" = 1.746"
equation "\"Угол_зацепления\" = 20deg"
equation "\"Зазор_профиля_зуба\" = 0.25"
equation "\"Радиус_закругления_зуба\" = 0.2386"
equation "\"Диаметр_головки\" = 33.17505"
equation "\"Диаметр_впадин\" = 25.31805"
equation "\"Основной_диаметр\" = 27.89196"
equation "\"Средний_диаметр\" = 29.682"
equation "\"Ширина_грани\" = 6"
equation "\"Коэффициент_смещения\" = 0.0003"
equation "\"Изменение_высоты_головки_зуба\" = 0"
equation "\"Окружной_шаг\" = 5.48522"
equation "\"Общий_сдвиг_инструмента\" = 0.00052"
equation "\"Внутренний\" = 0"
